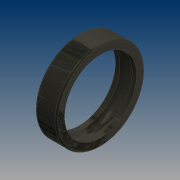
# Autodesk Inventor part: Outer Ring
Saved by Autodesk Inventor 2014 (Build 180170000, 170)
## iProperties
Created: 2021-03-19
Part Number: Outer Ring
Material: Lead
Document SubType Name: Modeling
Designer: Think Station
Density: 11.37 g/cm^3
Appearance: Gunmetal
Author: Think Station
Autodesk Inventor part; units mm, degrees
ref_plane "YZ Plane" through (0, 0, 0) normal (1, 0, 0) x (0, 1, 0)
ref_plane "XZ Plane" through (0, 0, 0) normal (0, 1, 0) x (-1, 0, 0)
ref_plane "XY Plane" through (0, 0, 0) normal (0, 0, 1) x (1, 0, 0)
sketch "Sketch1" plane through (0, 0, 0) normal (0, 0, 1) x (1, 0, 0)
  line L0 (-15.5, 65) -> (15.5, 65)
  line L1 (15.5, 65) -> (15.5, 53)
  line L2 (15.5, 53) -> (-15.5, 53)
  line L3 (-15.5, 53) -> (-15.5, 65)
  arc A0 (8.9443, 53) -> (-8.9443, 53) centre (0, 45) ccw
  line L4 (-21.7, 0) -> (21.7, 0) projected
  point P0 (0, 0)
  dimension "d0" = 31
  dimension "d1" = 12
  dimension "d2" = 53
  dimension "d3" = 15.5
  dimension "d4" = 8
  dimension "d5" = 12
  constraints: 8 end point, 2 parallel, 2 point on circle, 2 point on line, 1 centre point, 1 horizontal, 1 perpendicular, 1 vertical alignment
  measures "d0" distance between parallel lines of L1 L3
  measures "d1" distance of L0.end L1.end
  measures "d2" distance from line of point (0, 0) L2
  measures "d3" distance from line of L1 point (0, 0)
  measures "d4" distance from line of L2 A0.centre
  measures "d5" radius of A0
revolve "Revolution1" add sketch "Sketch1" angle 360 about axis through (-10, 0, 0) along (1, 0, 0) contours L0 L1 L2 A0 L3
fillet "Fillet1" radius 2.1 2 edges at (15.5, -65, 0) (-15.5, -65, 0)
body "Solid1"
